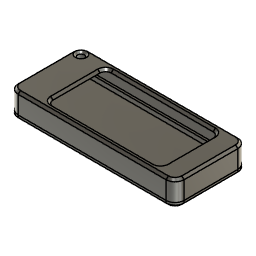
3D Design Workshop (Autodesk Fusion 360 design; units mm, degrees)
Autodesk Fusion 360 part; units mm, degrees
sketch "Sketch1" plane through (0, 0, 0) normal (0, 0, 1) x (1, 0, 0) in component "Face Piece"
  line L0 (-3, 0) -> (-69, 0)
  line L1 (-72, 3) -> (-72, 27)
  line L2 (-69, 30) -> (-3, 30)
  line L3 (0, 27) -> (0, 3)
  circle A0 centre (-2.5, 2.5) radius 1.5
  circle A1 centre (-2.5, 27.5) radius 1.5
  circle A2 centre (-69.5, 2.5) radius 1.5
  circle A3 centre (-69.5, 27.5) radius 1.5
  arc A4 (-69, 30) -> (-72, 27) centre (-69, 27) ccw
  arc A5 (-72, 3) -> (-69, 0) centre (-69, 3) ccw
  arc A6 (-3, 0) -> (0, 3) centre (-3, 3) ccw
  arc A7 (0, 27) -> (-3, 30) centre (-3, 27) ccw
  arc A8 (1, 27) -> (-3, 31) centre (-3, 27) ccw
  line L4 (-69, 31) -> (-3, 31)
  arc A9 (-69, 31) -> (-73, 27) centre (-69, 27) ccw
  line L5 (-73, 3) -> (-73, 27)
  arc A10 (-73, 3) -> (-69, -1) centre (-69, 3) ccw
  line L6 (-3, -1) -> (-69, -1)
  arc A11 (-3, -1) -> (1, 3) centre (-3, 3) ccw
  line L7 (1, 27) -> (1, 3)
  line L8 (-56.5, 28) -> (-11, 28)
  line L9 (-8.5, 25.5) -> (-8.5, 4.5)
  line L10 (-11, 2) -> (-56.5, 2)
  line L11 (-59, 4.5) -> (-59, 25.5)
  arc A12 (-56.5, 28) -> (-59, 25.5) centre (-56.5, 25.5) ccw
  arc A13 (-59, 4.5) -> (-56.5, 2) centre (-56.5, 4.5) ccw
  arc A14 (-11, 2) -> (-8.5, 4.5) centre (-11, 4.5) ccw
  arc A15 (-8.5, 25.5) -> (-11, 28) centre (-11, 25.5) ccw
  point P0 (-72, 0)
  dimension "d1" = 72
  dimension "d2" = 30
  dimension "d3" = 3
  dimension "d4" = 2.5
  dimension "d5" = 2.5
  dimension "d6" = 3
  dimension "d7" = 3
  dimension "d8" = 3
  dimension "d9" = 2.5
  dimension "d10" = 2.5
  dimension "d11" = 2.5
  dimension "d12" = 2.5
  dimension "d13" = 2.5
  dimension "d14" = 2.5
  dimension "d15" = 3
  dimension "d16" = -1
  dimension "d17" = 13
  dimension "d18" = 8.5
  dimension "d19" = 2
  dimension "d20" = 2
  dimension "d21" = 2.5
  constraint horizontal L0
  constraint vertical L1
  constraint horizontal L2
  constraint vertical L3
  constraint tangent L1 A4
  constraint tangent L2 A4
  constraint coincident P0 L0
  constraint coincident P0 L1
  constraint tangent L0 A5
  constraint tangent L1 A5
  constraint equal A4 A5
  constraint coincident origin L0
  constraint coincident origin L3
  constraint tangent L0 A6
  constraint tangent L3 A6
  constraint equal A4 A6
  constraint tangent L2 A7
  constraint tangent L3 A7
  constraint equal A4 A7
  constraint horizontal L8
  constraint vertical L9
  constraint horizontal L10
  constraint vertical L11
  constraint tangent L8 A12
  constraint tangent L11 A12
  constraint tangent L10 A13
  constraint tangent L11 A13
  constraint equal A12 A13
  constraint tangent L9 A14
  constraint tangent L10 A14
  constraint equal A12 A14
  constraint tangent L8 A15
  constraint tangent L9 A15
  constraint equal A12 A15
  measures "d1" distance of origin P0
  measures "d2" distance of L0 L2
  measures "d3" diameter of A0
  measures "d4" distance of L3 A0.centre
  measures "d5" distance of L0 A0.centre
  measures "d6" diameter of A1
  measures "d7" diameter of A2
  measures "d8" diameter of A3
  measures "d9" distance of L3 A1.centre
  measures "d10" distance of L2 A1.centre
  measures "d11" distance of L2 A3.centre
  measures "d12" distance of L1 A3.centre
  measures "d13" distance of L1 A2.centre
  measures "d14" distance of L0 A2.centre
  measures "d15" radius of A4
  measures "d17" distance of L1 L11
  measures "d18" distance of L3 L9
  measures "d19" distance of L2 L8
  measures "d20" distance of L0 L10
  measures "d21" radius of A12
extrude "Extrude1" add sketch "Sketch1" along normal blind 1 contours L0 L1 L2 L3 A4 A5 A6 A7 | A8 L4 A9 L5 A10 L6 A11 L7 makes body 1
extrude "Extrude2" add sketch "Sketch1" against normal blind 8 contours A8 L4 A9 L5 A10 L6 A11 L7 bodies 1
extrude "Extrude3" add sketch "Sketch1" along normal blind 1 contours A0 | A1 | A2 bodies 1
chamfer "Chamfer1" distance 1 angle 45 1 faces at (-67.0554, 11.1792, 1) on bodies 1
copy_body "CutPasteBodies1" bodies 1 removing the originals makes body 2 in component "Face Piece"
move_body "Move1" bodies 2 to x (1, 0, 0) y (0, 1, 0) z (0, 0, 1) at (0, 0, 8) in component "Face Piece"
sketch "Sketch1 (2)" plane through (0, 0, 0) normal (0, 0, 1) x (1, 0, 0) in component "Back Piece"
  line L0 (-32.6099, 13.4549) -> (33.3901, 13.4549)
  line L1 (36.3901, 10.4549) -> (36.3901, -13.5451)
  line L2 (33.3901, -16.5451) -> (-32.6099, -16.5451)
  line L3 (-35.6099, -13.5451) -> (-35.6099, 10.4549)
  circle A0 centre (-33.1099, 10.9549) radius 1.25
  arc A1 (-32.6099, 13.4549) -> (-35.6099, 10.4549) centre (-32.6099, 10.4549) ccw
  arc A2 (-35.6099, -13.5451) -> (-32.6099, -16.5451) centre (-32.6099, -13.5451) ccw
  arc A3 (33.3901, -16.5451) -> (36.3901, -13.5451) centre (33.3901, -13.5451) ccw
  arc A4 (36.3901, 10.4549) -> (33.3901, 13.4549) centre (33.3901, 10.4549) ccw
  arc A5 (-32.6099, 14.4549) -> (-36.6099, 10.4549) centre (-32.6099, 10.4549) ccw
  line L4 (-36.6099, -13.5451) -> (-36.6099, 10.4549)
  arc A6 (-36.6099, -13.5451) -> (-32.6099, -17.5451) centre (-32.6099, -13.5451) ccw
  line L5 (33.3901, -17.5451) -> (-32.6099, -17.5451)
  arc A7 (33.3901, -17.5451) -> (37.3901, -13.5451) centre (33.3901, -13.5451) ccw
  line L6 (37.3901, 10.4549) -> (37.3901, -13.5451)
  arc A8 (37.3901, 10.4549) -> (33.3901, 14.4549) centre (33.3901, 10.4549) ccw
  line L7 (-32.6099, 14.4549) -> (33.3901, 14.4549)
  arc A9 (35.3901, 10.4549) -> (33.3901, 12.4549) centre (33.3901, 10.4549) ccw
  line L8 (-32.6099, 12.4549) -> (33.3901, 12.4549)
  arc A10 (-32.6099, 12.4549) -> (-34.6099, 10.4549) centre (-32.6099, 10.4549) ccw
  line L9 (-34.6099, -13.5451) -> (-34.6099, 10.4549)
  arc A11 (-34.6099, -13.5451) -> (-32.6099, -15.5451) centre (-32.6099, -13.5451) ccw
  line L10 (33.3901, -15.5451) -> (-32.6099, -15.5451)
  arc A12 (33.3901, -15.5451) -> (35.3901, -13.5451) centre (33.3901, -13.5451) ccw
  line L11 (35.3901, 10.4549) -> (35.3901, -13.5451)
  circle A13 centre (-33.1099, -14.0451) radius 1.25
  circle A14 centre (33.8901, 10.9549) radius 1.25
  circle A15 centre (33.8901, -14.0451) radius 1.25
  point P0 (-35.6099, 13.4549)
  point P1 (36.3901, 13.4549)
  point P2 (-35.6099, -16.5451)
  dimension "d29" = 72
  dimension "d30" = 30
  dimension "d31" = 2.5
  dimension "d32" = 2.5
  dimension "d33" = 2.5
  dimension "d34" = 3
  dimension "d35" = -1
  dimension "d36" = 1
  dimension "d37" = 2.5
  dimension "d38" = 2.5
  dimension "d39" = 2.5
  constraint horizontal L0
  constraint vertical L1
  constraint horizontal L2
  constraint vertical L3
  constraint coincident P0 L0
  constraint coincident P0 L3
  constraint tangent L0 A1
  constraint tangent L3 A1
  constraint coincident P2 L2
  constraint coincident P2 L3
  constraint tangent L2 A2
  constraint tangent L3 A2
  constraint equal A1 A2
  constraint tangent L1 A3
  constraint tangent L2 A3
  constraint equal A1 A3
  constraint coincident P1 L0
  constraint coincident P1 L1
  constraint tangent L0 A4
  constraint tangent L1 A4
  constraint equal A1 A4
  measures "d29" distance of P0 P1
  measures "d30" distance of P0 P2
  measures "d31" diameter of A0
  measures "d32" distance of L0 A0.centre
  measures "d33" distance of L3 A0.centre
  measures "d34" radius of A1
  measures "d37" diameter of A13
  measures "d38" diameter of A14
  measures "d39" diameter of A15
extrude "Extrude1'" add sketch "Sketch1 (2)" against normal blind 2 separate body contours L0 L1 L2 L3 A1 A2 A3 A4 | A5 L4 A6 L5 A7 L6 A8 L7 | A9 L8 A10 L9 A11 L10 A12 L11 | A13 | A14 | A15 makes body 3 in component "Back Piece"
extrude "Extrude2'" add sketch "Sketch1 (2)" along normal blind 2 contours L0 L1 L2 L3 A1 A2 A3 A4 bodies 3 in component "Back Piece"
chamfer "Chamfer1'" distance 1 angle 45 1 faces at (11.6216, 2.4987, -2) on bodies 3 in component "Back Piece"
sketch "Sketch2" plane through (0, 14.4549, 0) normal (0, 1, 0) x (-1, 0, 0) in component "Back Piece"
  line L0 (-33.3901, -1) -> (32.6099, -1)
  line L1 (32.6099, -1) -> (32.6099, 0)
  line L2 (32.6099, 0) -> (-33.3901, 0)
  line L3 (-33.3901, 0) -> (-33.3901, -1)
  line L4 (-0.3901, -1) -> (-0.3901, 0)
  line L5 (-0.3901, -1) -> (-4.1901, -1)
  line L6 (-4.3901, -0.8) -> (-4.3901, -0.2)
  line L7 (-4.1901, 0) -> (-0.3901, 0)
  line L8 (-0.3901, 0) -> (-0.3901, -1)
  line L9 (-0.3901, -1) -> (3.4099, -1)
  line L10 (3.6099, -0.8) -> (3.6099, -0.2)
  line L11 (3.4099, 0) -> (-0.3901, 0)
  line L12 (-0.3901, 0) -> (-0.3901, -1)
  arc A0 (3.4099, -1) -> (3.6099, -0.8) centre (3.4099, -0.8) ccw
  arc A1 (3.6099, -0.2) -> (3.4099, 0) centre (3.4099, -0.2) ccw
  arc A2 (-4.1901, 0) -> (-4.3901, -0.2) centre (-4.1901, -0.2) ccw
  arc A3 (-4.3901, -0.8) -> (-4.1901, -1) centre (-4.1901, -0.8) ccw
  dimension "d45" = 4
  dimension "d46" = 4
  dimension "d47" = 0.2
  dimension "d48" = 0.2
  constraint midpoint L0 L4.start
  constraint midpoint L2 L4.end
  constraint horizontal L5
  constraint vertical L6
  constraint horizontal L7
  constraint vertical L8
  constraint horizontal L9
  constraint vertical L10
  constraint horizontal L11
  constraint vertical L12
  constraint tangent L9 A0
  constraint tangent L10 A0
  constraint tangent L10 A1
  constraint tangent L11 A1
  constraint equal A0 A1
  constraint tangent L6 A2
  constraint tangent L7 A2
  constraint equal A0 A2
  constraint tangent L5 A3
  constraint tangent L6 A3
  measures "d45" distance of L10 L12
  measures "d46" distance of L6 L12
  measures "d47" radius of A0
  measures "d48" radius of A3
extrude "Extrude3'" cut sketch "Sketch2" against normal blind 1.5 contours L0 L2 L4 L5 L6 L7 L8 L12 A2 A3 | L0 L2 L4 L8 L9 L10 L11 L12 A0 A1 bodies 3 in component "Back Piece"
move_body "Move1'" bodies 3 to x (1, 0, 0) y (0, 1, 0) z (0, 0, 1) at (-36.3901, 16.5451, 0) in component "Back Piece"
component "Face Piece" placed x (1, 0, 0) y (0, 1, 0) z (0, 0, 1) at (0, 0, 0)
component "Back Piece" placed x (1, 0, 0) y (0, 1, 0) z (0, 0, 1) at (0, 0, 0)
named bodies: "Face Piece", "Back Plate"
